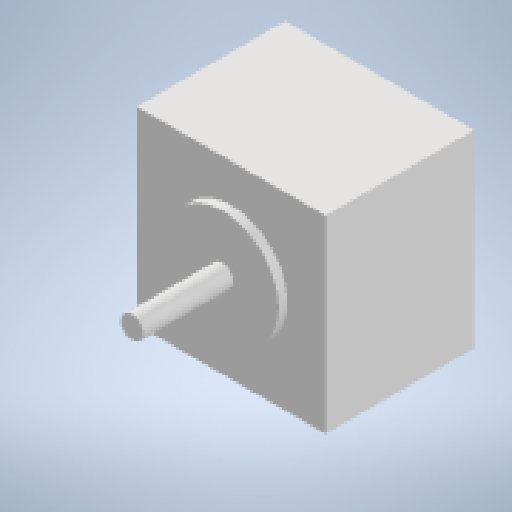
# Autodesk Inventor part: motor_sample
Saved by Autodesk Inventor 2023 (Build 270158000, 158)
## iProperties
Created: 2022-09-15
Part Number: motor_sample
Material: Generic
Document SubType Name: Modeling
Designer: simon
Density: 1 g/cm^3
Appearance: Default
Author: simon
Autodesk Inventor part; units mm, degrees
ref_plane "YZ Plane" through (0, 0, 0) normal (1, 0, 0) x (0, 1, 0)
ref_plane "XZ Plane" through (0, 0, 0) normal (0, 1, 0) x (-1, 0, 0)
ref_plane "XY Plane" through (0, 0, 0) normal (0, 0, 1) x (1, 0, 0)
sketch "Sketch1" plane through (0, 0, 0) normal (0, 0, 1) x (1, 0, 0)
  line L0 (16.5, 21.5) -> (16.5, 26.5) projected
  line L1 (16.5, 26.5) -> (16.5, 76.5) projected
  line L2 (16.5, 76.5) -> (26.5, 76.5) projected
  line L3 (26.5, 76.5) -> (26.5, 129.5) projected
  line L4 (26.5, 129.5) -> (-26.5, 129.5) projected
  line L5 (-26.5, 129.5) -> (-26.5, 76.5) projected
  line L6 (-26.5, 76.5) -> (-16.5, 76.5) projected
  line L7 (-16.5, 76.5) -> (-16.5, 26.5) projected
  line L8 (-16.5, 26.5) -> (-16.5, 21.5) projected
  line L9 (-16.5, 21.5) -> (-21.5, 21.5) projected
  line L10 (-21.5, 21.5) -> (-21.5, 11.5) projected
  line L11 (-21.5, 11.5) -> (-26.5, 11.5) projected
  line L12 (-26.5, 11.5) -> (-26.5, -11.5) projected
  line L13 (-26.5, -11.5) -> (-21.5, -11.5) projected
  line L14 (-21.5, -11.5) -> (-21.5, -21.5) projected
  line L15 (-21.5, -21.5) -> (-16.5, -21.5) projected
  line L16 (-16.5, -21.5) -> (-16.5, -26.5) projected
  line L17 (-16.5, -26.5) -> (-16.5, -76.5) projected
  line L18 (-16.5, -76.5) -> (-26.5, -76.5) projected
  line L19 (-26.5, -76.5) -> (-26.5, -129.5) projected
  line L20 (-26.5, -129.5) -> (26.5, -129.5) projected
  line L21 (26.5, -129.5) -> (26.5, -76.5) projected
  line L22 (26.5, -76.5) -> (16.5, -76.5) projected
  line L23 (16.5, -76.5) -> (16.5, -26.5) projected
  line L24 (16.5, -26.5) -> (16.5, -21.5) projected
  line L25 (16.5, -21.5) -> (21.5, -21.5) projected
  line L26 (21.5, -21.5) -> (21.5, -11.5) projected
  line L27 (21.5, -11.5) -> (26.5, -11.5) projected
  line L28 (26.5, -11.5) -> (26.5, 11.5) projected
  line L29 (26.5, 11.5) -> (21.5, 11.5) projected
  line L30 (21.5, 11.5) -> (21.5, 21.5) projected
  line L31 (21.5, 21.5) -> (16.5, 21.5) projected
  circle A0 centre (0, -103) radius 10.5 projected
  circle A1 centre (0, 103) radius 10.5 projected
  line L32 (-11.5, 26.5) -> (-11.5, 76.5) projected
  line L33 (-11.5, 76.5) -> (11.5, 76.5) projected
  line L34 (11.5, 76.5) -> (11.5, 26.5) projected
  line L35 (11.5, 26.5) -> (-11.5, 26.5) projected
  line L36 (11.5, -26.5) -> (11.5, -76.5) projected
  line L37 (11.5, -76.5) -> (-11.5, -76.5) projected
  line L38 (-11.5, -76.5) -> (-11.5, -26.5) projected
  line L39 (-11.5, -26.5) -> (11.5, -26.5) projected
  line L40 (-21, 21) -> (21, 21)
  line L41 (21, 21) -> (21, -21)
  line L42 (21, -21) -> (-21, -21)
  line L43 (-21, -21) -> (-21, 21)
  line L44 (-21, 21) -> (21, -21) construction
  line L45 (21, 21) -> (-21, -21) construction
  point P0 (0, 0)
  dimension "d0" = 42
  dimension "d1" = 42
  constraints: 12 end point, 2 midpoint, 2 parallel, 1 horizontal, 1 perpendicular
  measures "d0" distance of L41.end L42.end
  measures "d1" distance of L40.end L41.end
extrude "Extrusion1" add sketch "Sketch1" along normal blind 33 contours L40 L41 L42 L43
sketch "Sketch2" plane through (0, 0, 33) normal (0, 0, 1) x (1, 0, 0)
  circle A0 centre (0, 0) radius 12.5
  dimension "d4" = 25
  constraints: 1 centre point, 1 coincident
  measures "d4" diameter of A0
extrude "Extrusion2" add sketch "Sketch2" along normal blind 2
sketch "Sketch3" plane through (0, 0, 35) normal (0, 0, 1) x (1, 0, 0)
  circle A0 centre (0, 0) radius 2.5
  dimension "d7" = 5
  constraints: 1 centre point, 1 coincident
  measures "d7" diameter of A0
extrude "Extrusion3" add sketch "Sketch3" along normal blind 20
body "Solid1"
